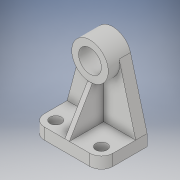
# Autodesk Inventor part: 示範三
Saved by Autodesk Inventor 2017 (Build 210142000, 142)
## iProperties
Part Number: 示範三
Material: 一般
Document SubType Name: Modeling
Designer: user01
Density: 1 g/cm^3
Appearance: 預設
Author: user01
Autodesk Inventor part; units mm, degrees
ref_plane "YZ Plane" through (0, 0, 0) normal (1, 0, 0) x (0, 1, 0)
ref_plane "XZ Plane" through (0, 0, 0) normal (0, 1, 0) x (-1, 0, 0)
ref_plane "XY Plane" through (0, 0, 0) normal (0, 0, 1) x (1, 0, 0)
sketch "草圖1" plane through (0, 0, 0) normal (0, 1, 0) x (-1, 0, 0)
  line L0 (0, 0) -> (-15, 0)
  line L1 (-15, 0) -> (-15, 20)
  line L2 (-15, 20) -> (0, 20)
  line L3 (0, 0) -> (0, -3.6184)
  line L4 (0, 0) -> (15, 0)
  line L5 (15, 0) -> (15, 20)
  line L6 (15, 20) -> (0, 20)
  dimension "d0" = 30
  dimension "d1" = 20
  constraints: 14 end point, 2 perpendicular, 2 symmetric about line, 1 horizontal, 1 vertical
  measures "d0" distance of L1.end L5.end
  measures "d1" distance of L0.end L1.end
extrude "擠出1" add sketch "草圖1" along normal blind 5
fillet "圓角1" radius 5 2 edges at (15, 2.5, 20) (-15, 2.5, 20)
sketch "草圖2" plane through (15, 0, 0) normal (0, 0, -1) x (-1, 0, 0)
  line L0 (15, 0) -> (15, 30)
  line L1 (30, 0) -> (0, 0) projected
  circle A0 centre (15, 30) radius 8
  circle A1 centre (15, 30) radius 5
  dimension "d5" = 30
  dimension "d6" = 16
  dimension "d7" = 10
  constraints: 2 centre point, 2 coincident, 2 end point, 1 vertical
  measures "d5" distance from line of L0.end L1
  measures "d6" diameter of A0
  measures "d7" diameter of A1
extrude "擠出2" add sketch "草圖2" against normal blind 10
sketch "草圖4" plane through (15, 0, 0) normal (0, 0, -1) x (-1, 0, 0)
  line L0 (0, 5) -> (30, 5) projected
  line L1 (0, 5) -> (7.274, 32.0756)
  circle A0 centre (15, 30) radius 8 projected
  line L2 (15, 22) -> (15, 5)
  line L3 (0, 5) -> (15, 5)
  line L4 (25, 5) -> (5, 5) projected
  arc A1 (7.274, 32.0756) -> (15, 22) centre (15, 30) ccw
  point P0 (15, 0)
  dimension "d14" = 15
  constraints: 6 end point, 4 point on circle, 1 centre point, 1 coincident, 1 collinear, 1 midpoint, 1 tangent
  measures "d14" distance from line of L2 L0.start
extrude "擠出3" add sketch "草圖4" against normal blind 5 contours L1 A0 L2 L0
sketch "草圖5" plane through (15, 0, 0) normal (0, 0, -1) x (-1, 0, 0)
  line L0 (30, 5) -> (15, 5)
  line L1 (15, 5) -> (15, 22.1541)
  line L2 (30, 5) -> (22.726, 32.0756)
  arc A0 (15, 22) -> (7.274, 32.0756) centre (15, 30) ccw projected
  arc A1 (15, 22) -> (22.726, 32.0756) centre (15, 30) ccw
  line L3 (15, 30) -> (15, 33.3003) construction
  line L4 (15, 5) -> (30, 5) projected
  point P0 (15, 0)
  dimension "d17" = 15
  constraints: 8 end point, 2 collinear, 2 point on circle, 1 centre point, 1 coincident, 1 concentric, 1 horizontal, 1 perpendicular, 1 point on line, 1 tangent, 1 vertical
  measures "d17" distance from line of L0.start L1
extrude "擠出4" add sketch "草圖5" against normal blind 5
sketch "草圖6" plane through (0, 0, 0) normal (1, 0, 0) x (0, 1, 0)
  line L0 (5, 20) -> (22, 10)
  line L1 (22, 5) -> (22, 10) projected
  line L2 (5, 20) -> (5, 5)
  line L3 (5, 5) -> (22, 5)
  line L4 (5, 5) -> (32.0756, 5) projected
  point P0 (0, 0)
  dimension "d20" = 15
  dimension "d21" = 17
  constraints: 6 end point, 1 collinear, 1 perpendicular, 1 point on line, 1 vertical
  measures "d20" distance of L0.start L2.end
  measures "d21" distance between parallel lines of L1 L2
extrude "擠出5" add sketch "草圖6" along normal mid plane 2
sketch "草圖8" plane through (0, 5, 0) normal (0, 1, 0) x (1, 0, 0)
  arc A0 (10, -20) -> (15, -15) centre (10, -15) ccw projected
  circle A1 centre (10, -15) radius 2.5
  point P0 (0, 0)
  dimension "d24" = 5
  constraints: 1 centre point, 1 coincident
  measures "d24" diameter of A1
extrude "擠出6" cut sketch "草圖8" against normal up to next
sketch "草圖9" plane through (0, 5, 0) normal (0, 1, 0) x (1, 0, 0)
  arc A0 (-15, -15) -> (-10, -20) centre (-10, -15) ccw projected
  circle A1 centre (-10, -15) radius 2.5
  point P0 (0, 0)
  dimension "d27" = 5
  constraints: 1 centre point, 1 coincident
  measures "d27" diameter of A1
extrude "擠出7" cut sketch "草圖9" against normal up to next
